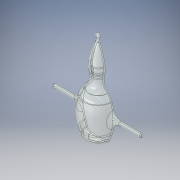
# Autodesk Inventor part: probenkammer-halbe
Saved by Autodesk Inventor 2017 (Build 210142000, 142)
## iProperties
Part Number: probenkammer-halbe
Material: Glas
Document SubType Name: Modeling
Designer: David
Density: 2.18 g/cm^3
Appearance: Klar
Author: David
Autodesk Inventor part; units mm, degrees
note: some values were not read from the file. Chosen so that the rebuilt part matches the saved one: edges of "Rundung2".
ref_plane "YZ Plane" through (0, 0, 0) normal (1, 0, 0) x (0, 1, 0)
ref_plane "XZ Plane" through (0, 0, 0) normal (0, 1, 0) x (-1, 0, 0)
ref_plane "XY Plane" through (0, 0, 0) normal (0, 0, 1) x (1, 0, 0)
sketch "Skizze1" plane through (0, 0, 0) normal (0, 1, 0) x (-1, 0, 0)
  arc A0 (0, 35.0724) -> (-1.0419, 33.4487) centre (0, 33.9263) ccw
  arc A1 (-0.9909, 31.3766) -> (-1.0419, 33.4487) centre (-3.4324, 32.3531) ccw
  arc A2 (-0.9909, 31.3766) -> (-3.7175, 21.3216) centre (40.9073, 14.6179) ccw
  arc A3 (-3.7175, 21.3216) -> (-3.5582, 18.4922) centre (3.1549, 20.2893) ccw
  arc A4 (-3.3558, 17.5192) -> (-3.5582, 18.4922) centre (-12.0594, 16.2165) ccw
  arc A5 (-5.175, 10.4495) -> (-3.1339, 16.0365) centre (-9.282, 15.1162) ccw
  arc A6 (-5.175, 10.4495) -> (-7.2883, 7.3009) centre (-0.2656, 4.8709) ccw
  line L0 (-3.1339, 16.0365) -> (-3.3558, 17.5192)
  line L1 (0, 35.0724) -> (0, -12.3679) construction
  arc A7 (-6.2573, -10.2854) -> (-3.7352, -12.2289) centre (-3.52, -9.3414) ccw
  arc A8 (-3.7352, -12.2289) -> (0, -12.3679) centre (0, 37.8899) ccw
  arc A9 (-8.6484, 3.8429) -> (-7.7357, 6.0077) centre (-24.6078, 11.8457) ccw
  line L2 (-7.7357, 6.0077) -> (-7.2883, 7.3009)
  arc A10 (-13.0922, 1.1) -> (-8.6484, 3.8429) centre (-13.0922, 6.0712) ccw construction
  line L3 (-13.0922, -1.1) -> (-13.0922, 1.1) construction
  line L4 (-13.0922, 1.1) -> (-23, 1.1)
  line L5 (-23, 1.1) -> (-23, -1.1) construction
  line L6 (-23, -1.1) -> (-13.0922, -1.1) construction
  arc A11 (-7.2883, 7.3009) -> (-7.2883, -7.3009) centre (13.8118, 0) ccw
  line L7 (-7.2883, -7.3009) -> (-7.2883, 7.3009) construction
  line L8 (13.8118, 0) -> (-23, 0) construction
  arc A12 (-6.2573, -10.2854) -> (-7.2883, -7.3009) centre (-2877.8088, -1000.5346) ccw
  line L9 (-23, 1.1) -> (-23, 0)
  line L10 (-23, 0) -> (-8.5157, 0)
  arc A13 (-2.9239, 21.2189) -> (-2.7854, 18.6991) centre (3.1549, 20.2893) ccw
  arc A14 (-2.5647, 17.6377) -> (-2.7854, 18.6991) centre (-12.0594, 16.2165) ccw
  line L11 (-2.5647, 17.6377) -> (-2.3427, 16.1549)
  arc A15 (-4.6465, 9.8489) -> (-2.3427, 16.1549) centre (-9.282, 15.1162) ccw
  arc A16 (-4.6465, 9.8489) -> (-6.5323, 7.0393) centre (-0.2656, 4.8709) ccw
  arc A17 (-6.5323, 7.0393) -> (-6.5323, -7.0393) centre (13.8118, 0) ccw
  arc A18 (-5.5011, -10.0246) -> (-6.5323, -7.0393) centre (-2877.8088, -1000.5346) ccw
  arc A19 (-5.5011, -10.0246) -> (-3.6757, -11.4312) centre (-3.52, -9.3414) ccw
  arc A20 (-3.6757, -11.4312) -> (0, -11.568) centre (0, 37.8899) ccw
  arc A21 (-0.2978, 30.9547) -> (0, 32.3531) centre (-3.4324, 32.3531) ccw construction
  arc A22 (-0.2978, 30.9547) -> (-2.9239, 21.2189) centre (40.9073, 14.6179) ccw
  line L12 (-13.0922, 1.1) -> (-13.0922, 0)
  arc A23 (0, 31.157) -> (-0.2978, 30.9547) centre (0, 30.8367) ccw
  line L13 (0, 31.157) -> (0, 35.0724)
  line L14 (0, -11.568) -> (0, -12.3679)
  point P0 (0, 0)
  point P1 (0, 30.2807)
  dimension "d91" = 2.2
  dimension "d117" = 0.8
  dimension "d137" = 23
  constraints: 49 point on circle, 28 end point, 24 centre point, 16 tangent, 3 point on line, 3 vertical, 2 collinear, 2 midpoint, 2 perpendicular, 1 horizontal, 1 parallel, 19 other
  measures "d91" distance of L4.end L5.end
  measures "d117" radial gap between concentric circles of A2 A22
  measures "d137" distance from line of point (0, 0) L5
revolve "Umdrehung1" add sketch "Skizze1" angle 360 about axis through (0, 0, 35.0724) along (0, 0, -1) contours L13 A23 A22 A13 A14 L11 A15 A16 A17 A18 A19 A20 L14 A8 A7 A12 A11 A6 A5 L0 A4 A3 A2 A1 A0
revolve "Umdrehung2" add sketch "Skizze1" angle 360 about axis through (-13.8118, 0, 0) along (1, 0, 0) contours L12 L10 L9 L4
sketch "Skizze6" plane through (13.0922, 0, 0) normal (-1, 0, 0) x (0, 0, 1)
  circle A0 centre (0, 0) radius 1.1 projected
  point P0 (0, 0)
extrude "Extrusion4" add sketch "Skizze6" along normal up to surface
fillet "Rundung2" radius 4 1 edges at (8.4665, 0.7772, 0.7784)
sketch "Skizze2" plane through (23, 0, 0) normal (1, 0, 0) x (0, 0, -1)
  circle A0 centre (0, 0) radius 0.5
  point P0 (0, 0)
  dimension "d122" = 1
  constraints: 1 centre point
  measures "d122" diameter of A0
extrude "Extrusion1" cut sketch "Skizze2" against normal up to surface (23 mm away)
mirror "Spiegeln3" about plane through (0, 0, 0) normal (1, 0, 0) of "Umdrehung2", "Extrusion4", "Rundung2", "Extrusion1"
sketch "Skizze7" plane through (0, 0, 0) normal (0, 1, 0) x (-1, 0, 0)
  line L0 (51.6998, 52.7341) -> (-44.4622, 52.7341)
  line L1 (-44.4622, 52.7341) -> (-44.4622, -26.9114)
  line L2 (-44.4622, -26.9114) -> (51.6998, -26.9114)
  line L3 (51.6998, -26.9114) -> (51.6998, 52.7341)
  point P0 (0, 0)
  constraints: 8 end point, 2 parallel, 1 horizontal, 1 perpendicular
extrude "Extrusion5" cut sketch "Skizze7" along normal blind 30.7
fillet "Rundung3" radius 0.5 2 edges at (23, -1.1, 0) (-23, -1.1, 0)
